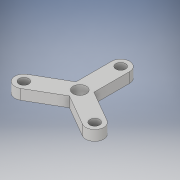
# Autodesk Inventor part: gearbox_secondary_gear_holder
Saved by Autodesk Inventor 2019 (Build 230136000, 136)
## iProperties
Created: 2019-12-24
Part Number: gearbox_secondary_gear_holder
Material: Типовые
Document SubType Name: Modeling
Designer: Петров Иван
Density: 1 g/cm^3
Appearance: По умолчанию
Author: Петров Иван
Autodesk Inventor part; units mm, degrees
ref_plane "YZ Plane" through (0, 0, 0) normal (1, 0, 0) x (0, 1, 0)
ref_plane "XZ Plane" through (0, 0, 0) normal (0, 1, 0) x (-1, 0, 0)
ref_plane "XY Plane" through (0, 0, 0) normal (0, 0, 1) x (1, 0, 0)
sketch "Эскиз1" plane through (0, 0, 0) normal (0, 1, 0) x (-1, 0, 0)
  point P0 (0, 0)
sketch "Эскиз2" plane through (0, 0, 0) normal (0, 1, 0) x (-1, 0, 0)
  line L0 (0, 0) -> (0, -16)
  circle A0 centre (0, -16) radius 1.9
  circle A1 centre (0, 0) radius 2.6
  line L1 (0, 0) -> (0, -16) construction
  line L2 (-3.5, 0) -> (-3.5, -16)
  line L3 (3.5, -16) -> (3.5, 0)
  arc A2 (3.5, 0) -> (-3.5, 0) centre (0, 0) ccw
  arc A3 (-3.5, -16) -> (3.5, -16) centre (0, -16) ccw
  point P0 (0, -8)
  dimension "d0" = 16
  dimension "d1" = 3.8
  dimension "d2" = 5.2
  dimension "d3" = 7
  constraints: 10 end point, 4 centre point, 4 point on circle, 4 tangent, 2 coincident, 2 equal length, 1 midpoint, 1 vertical
  measures "d0" distance of L0.start L0.end
  measures "d1" diameter of A0
  measures "d2" diameter of A1
  measures "d3" diameter of A3
extrude "Выдавливание1" add sketch "Эскиз2" along normal blind 4
pattern_circular "Круговой массив1" count 3 over 360 about axis through (0, 0, 0) along (0, 1, 0) of "Выдавливание1"
